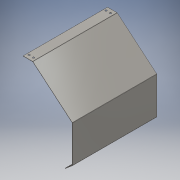
# Autodesk Inventor part: MC Part3
Saved by Autodesk Inventor 2016 (Build 200138000, 138)
## iProperties
Created: 2017-10-24
Part Number: MC Part3
Material: Steel, Mild
Document SubType Name: Sheet Metal
Designer: m207653
Density: 7.85 g/cm^3
Sheet Metal Rule: ms steel
Appearance: Semi-Polished
Flat Pattern Width: 57 cm
Flat Pattern Length: 72.8332 cm
Flat Pattern Area: 4151.49 cm^2
Sheet Metal Width: 570.000 mm
Sheet Metal Length: 728.332 mm
Sheet Metal Area: 415149.004 mm^2
Author: m207653
Autodesk Inventor part; units mm, degrees
ref_plane "YZ Plane" through (0, 0, 0) normal (1, 0, 0) x (0, 1, 0)
ref_plane "XZ Plane" through (0, 0, 0) normal (0, 1, 0) x (-1, 0, 0)
ref_plane "XY Plane" through (0, 0, 0) normal (0, 0, 1) x (1, 0, 0)
sketch "Sketch1" plane through (0, 0, 0) normal (1, 0, 0) x (0, 1, 0)
  line L0 (0, 0) -> (570, 0)
  line L1 (0, 0) -> (0, 251)
  line L2 (0, 251) -> (570, 251)
  line L3 (570, 251) -> (570, 0)
  dimension "d0" = 570
  dimension "d1" = 251
  measures "d0" distance of L0.start L0.end
  measures "d1" distance of L0.start L1.end
extrude "Plate1" add sketch "Sketch1" along normal blind 1.6
sketch "Sketch2" plane through (0.5715, 0, 249.7743) normal (0.6427876, 0, 0.7660444) x (0, -1, 0)
  line L0 (-570, 0) -> (0, 0)
  line L1 (0, 0) -> (0, 350)
  line L2 (0, 350) -> (-570, 350)
  line L3 (-570, 350) -> (-570, 0)
  constraints: 6 end point, 1 horizontal, 1 perpendicular, 1 vertical
edge flange "Flange1" height 350 angle -50 thickness 1.6 bend radius 1.6 thickness toward (0.6427876, 0, 0.7660444) relief straight relief width 1.6 relief depth 0.8 edges at (1.6, 285, 251) wall of the first edge with corners at (0.5715, 570, 249.7743) (0.5715, 0, 249.7743) (-267.544, 0, 474.75) (-267.544, 570, 474.75)
bend "Bend1"
corner "Corner1"
sketch "Sketch3" plane through (-266.5156, 0, 474.3757) normal (0, 0, 1) x (0, -1, 0)
  line L0 (-570, 0) -> (0, 0)
  line L1 (0, 0) -> (0, 65)
  line L2 (0, 65) -> (-570, 65)
  line L3 (-570, 65) -> (-570, 0)
  constraints: 6 end point, 1 horizontal, 1 perpendicular, 1 vertical
edge flange "Flange2" height 65 angle -40 thickness 1.6 bend radius 1.6 thickness toward (0, 0, 1) relief straight relief width 1.6 relief depth 0.8 edges at (-266.5156, 285, 475.9757) wall of the first edge with corners at (-266.5156, 570, 474.3757) (-266.5156, 0, 474.3757) (-331.5156, 0, 474.3757) (-331.5156, 570, 474.3757)
bend "Bend2"
corner "Corner2"
sketch "Sketch4" plane through (0.5715, 570, 1.2257) normal (0.6427876, 0, -0.7660444) x (0, -1, 0)
  line L0 (570, 0) -> (0, 0)
  line L1 (0, 0) -> (0, -65)
  line L2 (0, -65) -> (570, -65)
  line L3 (570, -65) -> (570, 0)
  constraints: 6 end point, 1 horizontal, 1 perpendicular, 1 vertical
edge flange "Flange3" height 65 angle -50 thickness 1.6 bend radius 1.6 thickness toward (0.6427876, 0, -0.7660444) relief straight relief width 1.6 relief depth 0.8 edges at (1.6, 285, 0) wall of the first edge with corners at (0.5715, 0, 1.2257) (0.5715, 570, 1.2257) (-49.2213, 570, -40.5555) (-49.2213, 0, -40.5555)
bend "Bend3"
corner "Corner3"
sketch "Sketch5" plane through (-331.5156, 0, 475.9757) normal (0, 0, 1) x (1, 0, 0)
  line L0 (0, 570) -> (0, 0) projected
  line L1 (0, 570) -> (60, 570)
  line L2 (63.8353, 570) -> (0, 570) projected
  line L3 (60, 570) -> (60, 0)
  line L4 (63.8353, 0) -> (0, 0) projected
  line L5 (60, 0) -> (0, 0)
  line L6 (0, 0) -> (0, 570)
  circle A0 centre (45, 545) radius 6
  circle A1 centre (15, 545) radius 6
  circle A2 centre (45, 25) radius 6
  circle A3 centre (15, 25) radius 6
  point P0 (331.5156, 0)
  dimension "d33" = 60
  dimension "d34" = 12
  dimension "d35" = 12
  dimension "d36" = 15
  dimension "d37" = 15
  dimension "d38" = 25
  dimension "d39" = 25
  dimension "d40" = 12
  dimension "d41" = 12
  dimension "d42" = 25
  dimension "d43" = 25
  constraints: 8 end point, 4 centre point, 2 point on line, 1 collinear, 1 horizontal, 1 perpendicular
  measures "d33" distance of L0.start L1.end
  measures "d34" diameter of A0
  measures "d35" diameter of A1
  measures "d36" distance from line of L3 A0.centre
  measures "d37" distance from line of L0 A1.centre
  measures "d38" distance from line of L1 A0.centre
  measures "d39" distance from line of L1 A1.centre
  measures "d40" diameter of A2
  measures "d41" diameter of A3
  measures "d42" distance from line of L4 A2.centre
  measures "d43" distance from line of L4 A3.centre
hole "Hole1" at (-286.5156, 545, 475.9757) at (-316.5156, 545, 475.9757) at (-286.5156, 25, 475.9757) at (-316.5156, 25, 475.9757) direction (0, 0, -1) diameter 12 end through all
sketch "Sketch6" plane through (-48.1929, 0, -41.7812) normal (0.6427876, 0, -0.7660444) x (-0.7660444, 0, -0.6427876)
  line L0 (0, 0) -> (0, 570) projected
  line L1 (0, 0) -> (-60, 0)
  line L2 (-63.5078, 0) -> (0, 0) projected
  line L3 (-60, 0) -> (-60, 570)
  line L4 (-63.5078, 570) -> (0, 570) projected
  line L5 (-60, 570) -> (0, 570)
  line L6 (0, 570) -> (0, 0)
  circle A0 centre (-45, 25) radius 6
  circle A1 centre (-15, 25) radius 6
  circle A2 centre (-45, 545) radius 6
  circle A3 centre (-15, 545) radius 6
  point P0 (-63.7743, 0)
  dimension "d51" = 60
  dimension "d52" = 12
  dimension "d53" = 12
  dimension "d54" = 25
  dimension "d55" = 25
  dimension "d56" = 15
  dimension "d57" = 15
  dimension "d58" = 12
  dimension "d59" = 12
  dimension "d60" = 25
  dimension "d61" = 25
  constraints: 8 end point, 4 centre point, 2 point on line, 1 collinear, 1 horizontal, 1 perpendicular
  measures "d51" distance of L0.start L1.end
  measures "d52" diameter of A0
  measures "d53" diameter of A1
  measures "d54" distance from line of L1 A0.centre
  measures "d55" distance from line of L1 A1.centre
  measures "d56" distance from line of L3 A0.centre
  measures "d57" distance from line of L0 A1.centre
  measures "d58" diameter of A2
  measures "d59" diameter of A3
  measures "d60" distance from line of L4 A2.centre
  measures "d61" distance from line of L4 A3.centre
hole "Hole2" at (-13.7209, 25, -12.8558) at (-36.7022, 25, -32.1394) at (-13.7209, 545, -12.8558) at (-36.7022, 545, -32.1394) direction (-0.6427876, 0, 0.7660444) diameter 12 end through all
equation "\"d49\" = Thickness"
equation "\"d67\" = Thickness"
equation "\"d3\" = BendReliefWidth"
equation "\"d4\" = BendReliefDepth"
equation "\"d5\" = MinimumRemnant"
equation "\"d6\" = BendRadius"
equation "\"d9\" = BendRadius"
equation "\"d10\" = CornerReliefSize"
equation "\"d11\" = GapSize"
equation "\"d12\" = JacobiRadiusSize"
equation "\"d13\" = BendReliefWidth"
equation "\"d14\" = BendReliefDepth"
equation "\"d15\" = MinimumRemnant"
equation "\"d16\" = BendRadius"
equation "\"d19\" = BendRadius"
equation "\"d20\" = CornerReliefSize"
equation "\"d21\" = GapSize"
equation "\"d22\" = JacobiRadiusSize"
equation "\"d23\" = BendReliefWidth"
equation "\"d24\" = BendReliefDepth"
equation "\"d25\" = MinimumRemnant"
equation "\"d26\" = BendRadius"
equation "\"d29\" = BendRadius"
equation "\"d30\" = CornerReliefSize"
equation "\"d31\" = GapSize"
equation "\"d32\" = JacobiRadiusSize"
equation "\"BendRadius\" = Thickness"
equation "\"BendReliefWidth\" = Thickness"
equation "\"BendReliefDepth\" = 0.5 * Thickness"
equation "\"CornerReliefSize\" = 4 * Thickness"
equation "\"MinimumRemnant\" = 2 * Thickness"
equation "\"TransitionRadius\" = BendRadius"
equation "\"JacobiRadiusSize\" = BendRadius"
equation "\"GapSize\" = Thickness"
equation "\"d2\" = BendRadius"
equation "\"Thickness\" = 1.6"
body "Solid1"
